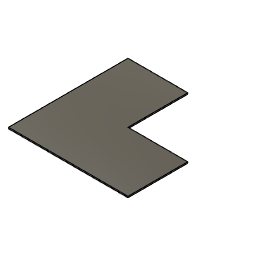
_SandwichPlate.160f049a-144e-4294-9e80-26d01a661236 (Autodesk Fusion 360 design; units mm, degrees)
Autodesk Fusion 360 part; units mm, degrees
sketch "Sketch1" plane through (0, 0, 0) normal (0, 0, 1) x (1, 0, 0)
  line L0 (0, 0) -> (0, 609.6)
  line L1 (0, 609.6) -> (304.8, 609.6)
  line L2 (304.8, 609.6) -> (304.8, 304.8)
  line L3 (304.8, 304.8) -> (609.6, 304.8)
  line L4 (609.6, 304.8) -> (609.6, 0)
  line L5 (609.6, 0) -> (0, 0)
  dimension "d1" = 304.8
  dimension "d2" = 609.6
  dimension "d3" = 304.8
  dimension "d4" = 609.6
  constraint coincident L0.start L5.end
  constraint vertical L0
  constraint perpendicular L0 L1
  constraint perpendicular L1 L2
  constraint perpendicular L2 L3
  constraint perpendicular L1 L4
  constraint perpendicular L0 L5
  measures "d1" distance of L3.end L4.end
  measures "d2" distance of L0.start L0.end
  measures "d3" distance of L0.end L1.end
  measures "d4" distance of L0.start L4.end
extrude "Extrude1" add sketch "Sketch1" along normal blind 6.35
